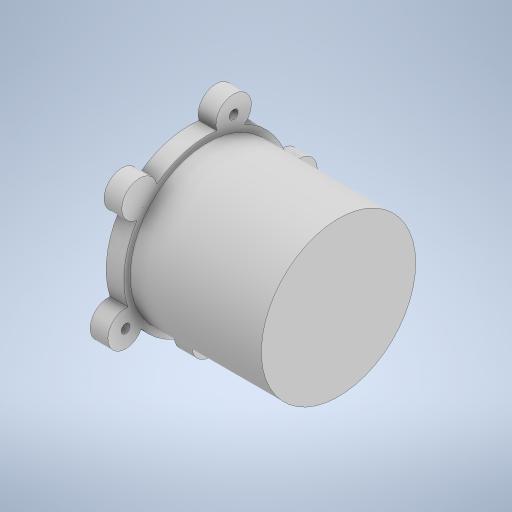
# Autodesk Inventor part: Двигатель ущербный
Saved by Autodesk Inventor 2023 (Build 270158000, 158)
## iProperties
Created: 2022-05-13
Part Number: Двигатель ущербный
Material: Типовые
Document SubType Name: Modeling
Designer: avkap
Density: 1 g/cm^3
Appearance: По умолчанию
Author: avkap
Autodesk Inventor part; units mm, degrees
ref_plane "YZ Plane" through (0, 0, 0) normal (1, 0, 0) x (0, 1, 0)
ref_plane "XZ Plane" through (0, 0, 0) normal (0, 1, 0) x (-1, 0, 0)
ref_plane "XY Plane" through (0, 0, 0) normal (0, 0, 1) x (1, 0, 0)
sketch "Эскиз1" plane through (0, 0, 0) normal (1, 0, 0) x (0, 1, 0)
  circle A0 centre (49.8341, -14.8513) radius 2.5
  circle A1 centre (-24.1951, 46.0282) radius 2.5
  circle A2 centre (-16.0232, -49.4698) radius 2.5
  arc A3 (42.0088, -21.0775) -> (46.6937, -5.3572) centre (49.8341, -14.8513) ccw
  arc A4 (37.4318, 28.4229) -> (25.3844, 39.5555) centre (35.2908, 38.1911) ccw
  arc A5 (-14.2733, 44.7803) -> (-28.7929, 37.1479) centre (-24.1951, 46.0282) ccw
  arc A6 (-46.4879, 6.9193) -> (-46.0344, -9.4779) centre (-51.9801, -1.4375) ccw
  arc A7 (41.8184, -21.4528) -> (42.2774, -21.4008) centre (35.2908, 38.1911) ccw
  arc A8 (59.6745, -16.6308) -> (-22.0673, 55.7992) centre (35.2908, 38.1911) ccw
  arc A9 (46.0698, -24.1158) -> (51.7554, -5.0376) centre (0, 0) ccw
  arc A10 (-27.3811, -38.2004) -> (-4.8121, -60.8851) centre (-16.0232, -49.4698) ccw
  arc A11 (8.6273, -51.2793) -> (9.7333, -51.0809) centre (0, 0) ccw
  arc A12 (-9.0725, -56.6592) -> (8.0019, -46.3138) centre (-0.2244, -51.9995) ccw
  arc A13 (-22.0629, -41.4997) -> (-9.0725, -56.6592) centre (-16.0232, -49.4698) ccw
  arc A14 (-18.3823, -48.6425) -> (-16.0232, -49.4698) centre (0, 0) ccw
  arc A15 (-29.7977, 54.3114) -> (-24.5001, -54.7746) centre (-51.9801, -1.4375) ccw
  arc A16 (-18.0553, -50.9259) -> (-16.0232, -49.4698) centre (-51.9801, -1.4375) ccw
  arc A17 (-46.0344, -9.4779) -> (-14.2733, 44.7803) centre (0, 0) ccw
  arc A18 (-28.7929, 37.1479) -> (-46.4879, 6.9193) centre (0, 0) ccw
  arc A19 (5.0161, -46.7316) -> (45.1354, 39.9476) centre (49.8341, -14.8513) ccw
  arc A20 (27.3279, 44.2401) -> (-14.9372, 49.8084) centre (0, 0) ccw
  arc A21 (29.9614, 36.433) -> (29.7793, 36.362) centre (49.8341, -14.8513) ccw
  arc A22 (29.927, 36.2405) -> (29.9614, 36.433) centre (-24.1951, 46.0282) ccw
  arc A23 (30.794, 47.1229) -> (-60.1153, 4.378) centre (-24.1951, 46.0282) ccw
  point P0 (-2.1659, -14.8513)
  dimension "d19" = 5
  dimension "d23" = 5
  dimension "d27" = 5
  dimension "d30" = 20
  dimension "d32" = 20
  dimension "d33" = 20
  constraints: 58 point on circle, 23 centre point, 8 coincident, 15 other
  measures "d19" diameter of A0
  measures "d23" diameter of A1
  measures "d27" diameter of A2
  measures "d30" diameter of A3
  measures "d32" diameter of A5
  measures "d33" diameter of A6
extrude "Выдавливание1" add sketch "Эскиз1" along normal blind 10 contours A0 A9 A3 | A0 A9 A3 A17 | A17 A6 A18 A5 | A17 A22 A21 A4 | A19 A11 A12 | A12 A13 A17 A19 | A12 A11 A19 A17
sketch "Эскиз2" plane through (10, 0, 0) normal (1, 0, 0) x (0, 0, -1)
  circle A0 centre (0, 0) radius 43.5
  dimension "d7" = 87
  constraints: 1 centre point, 1 coincident
  measures "d7" diameter of A0
extrude "Выдавливание2" add sketch "Эскиз2" along normal blind 74
sketch "Эскиз3" plane through (0, 0, 0) normal (-1, 0, 0) x (0, 0, 1)
  circle A0 centre (0, 0) radius 35
  dimension "d10" = 70
  constraints: 1 centre point, 1 coincident
  measures "d10" diameter of A0
extrude "Выдавливание3" add sketch "Эскиз3" along normal blind 5
sketch "Эскиз4" plane through (-5, 0, 0) normal (-1, 0, 0) x (0, 0, 1)
  circle A0 centre (0, 0) radius 16.5
  circle A1 centre (0, 0) radius 3
  dimension "d13" = 33
  dimension "d16" = 6
  constraints: 2 centre point, 2 coincident
  measures "d13" diameter of A0
  measures "d16" diameter of A1
extrude "Выдавливание4" add sketch "Эскиз4" along normal blind 10
